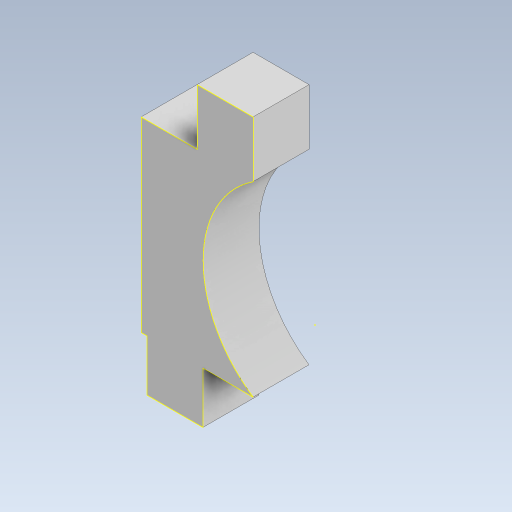
# Autodesk Inventor part: motorbase_2
Saved by Autodesk Inventor 2023 (Build 270158000, 158)
## iProperties
Created: 2023-04-18
Part Number: motorbase_2
Material: 一般
Document SubType Name: Modeling
Designer: Johnny Jou
Density: 1 g/cm^3
Appearance: 預設
Author: Johnny Jou
Autodesk Inventor part; units mm, degrees
ref_plane "YZ Plane" through (0, 0, 0) normal (1, 0, 0) x (0, 1, 0)
ref_plane "XZ Plane" through (0, 0, 0) normal (0, 1, 0) x (-1, 0, 0)
ref_plane "XY Plane" through (0, 0, 0) normal (0, 0, 1) x (1, 0, 0)
sketch "草圖1" plane through (0, 0, 0) normal (0, 0, 1) x (1, 0, 0)
  arc A0 (-3.3166, 5) -> (-3.3166, -5) centre (0, 0) ccw
  line L0 (-3.3166, -5) -> (-9.3166, -5)
  line L1 (-9.3166, -5) -> (-9.3166, 5)
  line L2 (-9.3166, 5) -> (-3.3166, 5)
  line L3 (-3.3166, 5) -> (-3.3166, -5) construction
  line L4 (-6.3166, -5) -> (-3.3166, -5)
  line L5 (-6.3166, 8) -> (-3.3166, 8)
  line L6 (-3.3166, 8) -> (-3.3166, 5)
  line L7 (-3.3166, 5) -> (-6.3166, 5)
  line L8 (-6.3166, 5) -> (-6.3166, 8)
  line L9 (-3.3166, -5) -> (3.3166, -5)
  arc A1 (-3.3166, 5) -> (-3.3166, -5) centre (0, 0) ccw
  arc A2 (3.3166, -5) -> (3.3166, 5) centre (0, 0) ccw
  line L10 (3.3166, 5) -> (-3.3166, 5)
  line L11 (-9.3166, -5) -> (-6, -5)
  line L12 (-6, -5) -> (-6, -7.7485)
  line L13 (-6, -7.7485) -> (-9, -7.7485)
  line L14 (-9, -7.7485) -> (-9, -5)
  point P0 (-6, 0)
  point P1 (-6, -6.3742)
  dimension "d0" = 6
  dimension "d3" = 3
  dimension "d4" = 3
  dimension "d5" = 10
  dimension "d6" = 3
  constraints: 30 end point, 7 point on circle, 6 horizontal, 6 parallel, 3 centre point, 3 perpendicular, 2 midpoint, 1 point on line, 1 vertical alignment, 4 other
  measures "d0" distance between parallel lines of L3 L1
  measures "d3" distance of L7.end L5.start
  measures "d4" distance of L5.start L5.end
  measures "d5" distance between parallel lines of L0 L2
  measures "d6" distance of L12.end L13.end
extrude "擠出1" add sketch "草圖1" along normal blind 3 contours A0 L0 L1 L2 | L2 L8 L5 L6 | L12 L13 L14 L0
sketch "草圖2" plane through (0, 0, 3) normal (0, 0, 1) x (1, 0, 0)
  line L0 (-6.3166, 8) -> (-6.3166, 5) projected
  line L1 (-6.3166, 5) -> (-9.3166, 5) projected
  line L2 (-9.3166, 5) -> (-9.3166, -5) projected
  line L3 (-9.3166, -5) -> (-9, -5) projected
  line L4 (-9, -5) -> (-9, -7.7485) projected
  line L5 (-9, -7.7485) -> (-6, -7.7485) projected
  line L6 (-6, -7.7485) -> (-6, -5) projected
  line L7 (-6, -5) -> (-3.3166, -5) projected
  arc A0 (-3.3166, 5) -> (-3.3166, -5) centre (0, 0) ccw projected
  line L8 (-3.3166, 5) -> (-3.3166, 8) projected
  line L9 (-3.3166, 8) -> (-6.3166, 8) projected
